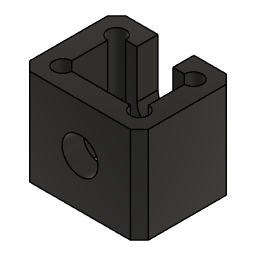
Prusa Expansion Joint (Autodesk Fusion 360 design; units mm, degrees)
Autodesk Fusion 360 part; units mm, degrees
note: some values were not read from the file. Set by a fixed rule: which sketch regions a step uses.
sketch "Sketch1" plane through (0, 0, 0) normal (0, 0, 1) x (1, 0, 0) in component "Prusa Expansion Joint"
  line L0 (-9.15, -8) -> (-0.75, -8)
  line L1 (0, -7.25) -> (0, -0.75)
  line L2 (-0.75, 0) -> (-9.15, 0)
  line L3 (-9.9, -0.75) -> (-9.9, -7.25)
  line L4 (-8.15, -6.25) -> (-1.75, -6.25)
  line L5 (-1.75, -6.25) -> (-1.75, -1.75)
  line L6 (-1.75, -1.75) -> (-8.15, -1.75)
  line L7 (-8.15, -1.75) -> (-8.15, -6.25)
  circle A0 centre (-1.75, -1.75) radius 0.75
  circle A1 centre (-8.15, -6.25) radius 0.75
  circle A2 centre (-8.15, -1.75) radius 0.75
  circle A3 centre (-1.75, -6.25) radius 0.75
  line L8 (-9.15, 0) -> (-9.9, -0.75)
  line L9 (-9.9, -7.25) -> (-9.15, -8)
  line L10 (0, -7.25) -> (-0.75, -8)
  line L11 (0, -0.75) -> (-0.75, 0)
  line L12 (0, -0.75) -> (0, 0) construction
  line L13 (0, 0) -> (-0.75, 0) construction
  dimension "d4" = 1.5
  dimension "d5" = 1.5
  dimension "d6" = 1.5
  dimension "d7" = 1.5
  dimension "d15" = 1.75
  dimension "d16" = 1.75
  dimension "d17" = 1.75
  dimension "d18" = 1.75
  dimension "d26" = 135
  dimension "d27" = 135
  dimension "d30" = 8
  dimension "d31" = 9.9
  dimension "d32" = 0.75
  constraint coincident L5.end L6.start
  constraint coincident L4.start L7.end
  constraint coincident L6.end L7.start
  constraint coincident L4.end L5.start
  constraint equal L4 L6
  constraint equal L5 L7
  constraint equal L1 L3
  constraint equal L0 L2
  constraint horizontal L0
  constraint horizontal L4
  constraint vertical L5
  constraint vertical L7
  constraint vertical L1
  constraint parallel L8 L10
  constraint equal L10 L11
  constraint parallel L9 L11
  constraint parallel L1 L12
  constraint perpendicular L12 L13
  constraint coincident L2.start L11.end
  constraint coincident L12.end L13.start
  measures "d4" diameter of A0
  measures "d5" diameter of A1
  measures "d6" diameter of A2
  measures "d7" diameter of A3
  measures "d15" distance of L1 L5
  measures "d16" distance of L3 L7
  measures "d17" distance of L2 L6
  measures "d18" distance of L0 L4
  measures "d26" angle of L2 L11
  measures "d27" angle of L0 L10
  measures "d30" distance of L2.end L0.start
  measures "d31" distance of L3.start L1.end
  measures "d32" horizontal distance of L2.end L3.start
extrude "Extrude1" add sketch "Sketch1" along normal blind 8 in component "Prusa Expansion Joint"
hole "Hole1" at (-4.95, -8, 4) direction (0, 1, 0) diameter 3 depth 8 tip angle 180 in component "Prusa Expansion Joint"
sketch "Sketch2" plane through (0, 0, 0) normal (0, 1, 0) x (1, 0, 0) in component "Prusa Expansion Joint"
  line L0 (-3.45, -4) -> (-6.45, -4)
  line L1 (-6.45, -4) -> (-6.45, -8)
  line L2 (-6.45, -8) -> (-3.45, -8)
  line L3 (-3.45, -8) -> (-3.45, -4)
  dimension "d33" = 3
  dimension "d34" = 4
  dimension "d35" = 4
  dimension "d36" = 3.45
  constraint horizontal L0
  constraint vertical L1
  constraint horizontal L2
  constraint vertical L3
  measures "d33" distance of L0.start L0.end
  measures "d34" distance of L0.start L2.end
  measures "d35" distance of L0 origin
  measures "d36" distance of L3 origin
extrude "Extrude2" cut sketch "Sketch2" against normal blind 1.75 in component "Prusa Expansion Joint"
component "Prusa Expansion Joint" placed x (1, 0, 0) y (0, 1, 0) z (0, 0, 1) at (0, 0, 0)
equation "d4 = ( 0.75 * 2 ) * 1 mm"
equation "d25 = ( 9.9 / 2 ) * 1 mm"
equation "d26 = 45 deg + 45 deg + 45 deg"
equation "d36 = ( ( 9.9 / 2 ) * 1 mm ) - 1.5 mm"
